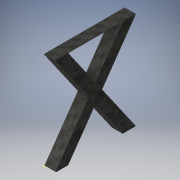
# Autodesk Inventor part: leg
Saved by Autodesk Inventor 2019 (Build 230136000, 136)
## iProperties
Created: 2019-07-26
Part Number: leg
Material: Steel
Document SubType Name: Modeling
Designer: Alex
Density: 7.85 g/cm^3
Appearance: Plate
Author: Alex
Autodesk Inventor part; units mm, degrees
ref_plane "YZ Plane" through (0, 0, 0) normal (1, 0, 0) x (0, 1, 0)
ref_plane "XZ Plane" through (0, 0, 0) normal (0, 1, 0) x (-1, 0, 0)
ref_plane "XY Plane" through (0, 0, 0) normal (0, 0, 1) x (1, 0, 0)
sketch "Sketch1" plane through (0, 0, 0) normal (1, 0, 0) x (0, 1, 0)
  line L0 (720, 0) -> (0, -502.4464)
  line L1 (0, -600) -> (720, -97.5536)
  line L2 (0, 0) -> (720, -502.4464)
  line L3 (720, -600) -> (0, -97.5536)
  line L4 (720, 0) -> (720, -97.5536)
  line L5 (720, -502.4464) -> (720, -600)
  line L6 (0, -600) -> (0, -502.4464)
  line L7 (0, -97.5536) -> (0, 0)
  dimension "d0" = 600
  dimension "d1" = 720
  dimension "d2" = 80
  dimension "d3" = 80
  constraints: 16 end point, 5 equal length, 1 vertical
  measures "d0" distance of L0.start L3.start
  measures "d1" distance of L3.start L1.start
  measures "d2" distance between parallel lines of L1 L0
  measures "d3" distance between parallel lines of L3 L2
sketch "Sketch2" plane through (0, 0, 0) normal (1, 0, 0) x (0, 1, 0)
  point P0 (0, 0)
extrude "Extrusion1" add sketch "Sketch1" along normal blind 80
fillet "Fillet1" radius 5 1 edges at (40, 360, -251.2232)
fillet "Fillet2" radius 5 1 edges at (40, 429.8966, -300)
fillet "Fillet3" radius 5 1 edges at (40, 360, -348.7768)
fillet "Fillet4" radius 5 1 edges at (40, 290.1034, -300)
sketch "Sketch3" plane through (80, 0, 0) normal (1, 0, 0) x (0, 0, -1)
  line L0 (502.4464, 720) -> (600, 720) projected
  line L1 (0, 723) -> (600, 723)
  line L2 (600, 723) -> (600, 720)
  line L3 (600, 720) -> (0, 720)
  line L4 (0, 720) -> (0, 723)
  point P0 (0, 0)
  dimension "d10" = 600
  dimension "d11" = 3
  constraints: 8 end point, 2 parallel, 1 horizontal, 1 perpendicular
  measures "d10" distance of L0.end L3.end
  measures "d11" distance between parallel lines of L1 L3
extrude "Extrusion2" add sketch "Sketch3" against normal blind 80
fillet "Fillet5" radius 5 1 edges at (40, 0, 0)
fillet "Fillet6" radius 5 1 edges at (40, 723, 0)
fillet "Fillet7" radius 5 1 edges at (40, 723, -600)
fillet "Fillet8" radius 5 1 edges at (40, 0, -600)
body "Solid1"
